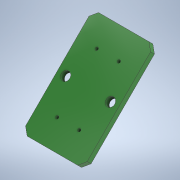
# Autodesk Inventor part: Button Module
Saved by Autodesk Inventor 2020 (Build 240168000, 168)
## iProperties
Created: 2021-01-14
Part Number: Button Module
Material: Generic
Document SubType Name: Modeling
Designer: Luke
Density: 1 g/cm^3
Appearance: Default
Author: Luke
Autodesk Inventor part; units mm, degrees
ref_plane "YZ Plane" through (0, 0, 0) normal (1, 0, 0) x (0, 1, 0)
ref_plane "XZ Plane" through (0, 0, 0) normal (0, 1, 0) x (-1, 0, 0)
ref_plane "XY Plane" through (0, 0, 0) normal (0, 0, 1) x (1, 0, 0)
ref_plane "Work Plane1" through (10.7635, -28.1998, -30.3509) normal (0, -0.7071068, -0.7071068) x (1, 0, 0)
sketch "Sketch1" plane through (10.7635, -28.1998, -30.3509) normal (0, -0.7071068, -0.7071068) x (1, 0, 0)
  line L0 (-49.4847, -25.5492) -> (-49.4847, -5.2292)
  arc A0 (-49.4466, -5.2292) -> (-49.5228, -5.2292) centre (-49.4847, -5.2292) ccw
  arc A1 (-49.5228, -25.5492) -> (-49.4466, -25.5492) centre (-49.4847, -25.5492) ccw
  line L1 (-49.4847, -5.2292) -> (-48.2147, -3.9592)
  arc A2 (-48.1878, -3.9861) -> (-48.2416, -3.9323) centre (-48.2147, -3.9592) ccw
  arc A3 (-49.5116, -5.2023) -> (-49.4578, -5.2561) centre (-49.4847, -5.2292) ccw
  line L2 (-48.2147, -3.9592) -> (-36.7847, -3.9592)
  arc A4 (-36.7847, -3.9973) -> (-36.7847, -3.9211) centre (-36.7847, -3.9592) ccw
  arc A5 (-48.2147, -3.9211) -> (-48.2147, -3.9973) centre (-48.2147, -3.9592) ccw
  line L3 (-36.7847, -3.9592) -> (-35.5147, -5.2292)
  arc A6 (-35.5416, -5.2561) -> (-35.4878, -5.2023) centre (-35.5147, -5.2292) ccw
  arc A7 (-36.7578, -3.9323) -> (-36.8116, -3.9861) centre (-36.7847, -3.9592) ccw
  line L4 (-35.5147, -5.2292) -> (-35.5147, -25.5492)
  arc A8 (-35.5528, -25.5492) -> (-35.4766, -25.5492) centre (-35.5147, -25.5492) ccw
  arc A9 (-35.4766, -5.2292) -> (-35.5528, -5.2292) centre (-35.5147, -5.2292) ccw
  line L5 (-35.5147, -25.5492) -> (-36.7847, -26.8192)
  arc A10 (-36.8116, -26.7923) -> (-36.7578, -26.8461) centre (-36.7847, -26.8192) ccw
  arc A11 (-35.4878, -25.5761) -> (-35.5416, -25.5223) centre (-35.5147, -25.5492) ccw
  line L6 (-36.7847, -26.8192) -> (-48.2147, -26.8192)
  arc A12 (-48.2147, -26.7811) -> (-48.2147, -26.8573) centre (-48.2147, -26.8192) ccw
  arc A13 (-36.7847, -26.8573) -> (-36.7847, -26.7811) centre (-36.7847, -26.8192) ccw
  line L7 (-48.2147, -26.8192) -> (-49.4847, -25.5492)
  arc A14 (-49.4578, -25.5223) -> (-49.5116, -25.5761) centre (-49.4847, -25.5492) ccw
  arc A15 (-48.2416, -26.8461) -> (-48.1878, -26.7923) centre (-48.2147, -26.8192) ccw
  circle A16 centre (-47.5797, -15.3892) radius 0.9525
  circle A17 centre (-37.4197, -15.3892) radius 0.9525
  arc A18 (-39.9597, -8.6572) -> (-39.9597, -9.2612) centre (-39.9597, -8.9592) ccw
  arc A19 (-39.9597, -9.2612) -> (-39.9597, -8.6572) centre (-39.9597, -8.9592) ccw
  arc A20 (-39.9597, -8.6572) -> (-39.9597, -9.2612) centre (-39.9597, -8.9592) ccw
  arc A21 (-39.9597, -9.2612) -> (-39.9597, -8.6572) centre (-39.9597, -8.9592) ccw
  arc A22 (-44.9597, -8.6572) -> (-44.9597, -9.2612) centre (-44.9597, -8.9592) ccw
  arc A23 (-44.9597, -9.2612) -> (-44.9597, -8.6572) centre (-44.9597, -8.9592) ccw
  arc A24 (-44.9597, -8.6572) -> (-44.9597, -9.2612) centre (-44.9597, -8.9592) ccw
  arc A25 (-44.9597, -9.2612) -> (-44.9597, -8.6572) centre (-44.9597, -8.9592) ccw
  arc A26 (-39.9597, -21.3572) -> (-39.9597, -21.9612) centre (-39.9597, -21.6592) ccw
  arc A27 (-39.9597, -21.9612) -> (-39.9597, -21.3572) centre (-39.9597, -21.6592) ccw
  arc A28 (-39.9597, -21.3572) -> (-39.9597, -21.9612) centre (-39.9597, -21.6592) ccw
  arc A29 (-39.9597, -21.9612) -> (-39.9597, -21.3572) centre (-39.9597, -21.6592) ccw
  arc A30 (-44.9597, -21.3572) -> (-44.9597, -21.9612) centre (-44.9597, -21.6592) ccw
  arc A31 (-44.9597, -21.9612) -> (-44.9597, -21.3572) centre (-44.9597, -21.6592) ccw
  arc A32 (-44.9597, -21.3572) -> (-44.9597, -21.9612) centre (-44.9597, -21.6592) ccw
  arc A33 (-44.9597, -21.9612) -> (-44.9597, -21.3572) centre (-44.9597, -21.6592) ccw
  point P0 (-39.9597, -21.9612)
  point P1 (-39.9597, -21.3572)
  point P2 (-39.9597, -9.2612)
  point P3 (-39.9597, -8.6572)
  point P4 (-48.2147, -26.8192)
  point P5 (-36.7847, -26.8192)
  point P6 (-35.5147, -25.5492)
  point P7 (-35.5147, -5.2292)
  point P8 (-36.7847, -3.9592)
  point P9 (-44.9597, -9.2612)
  point P10 (-44.9597, -8.6572)
  point P11 (-44.9597, -21.9612)
  constraints: 64 point on circle, 34 centre point, 16 end point
extrude "Extrusion1" add sketch "Sketch1" along normal blind 1.23 contours L0 L1 L2 L3 L4 L5 L6 L7
ref_plane "Work Plane2" through (-31.7362, -24.5021, -34.0485) normal (1, 0, 0) x (0, -0.7071068, -0.7071068)
ref_plane "Work Plane3" through (-26.0212, -17.3179, -41.2327) normal (0, 0.7071068, -0.7071068) x (-1, 0, 0)
ref_plane "Work Plane4" through (-37.4512, -10.1054, -50.1847) normal (0, 0, -1) x (1, 0, 0)
ref_plane "Work Plane5" through (-26.0212, -17.3179, -41.2327) normal (0, 0.7071068, -0.7071068) x (-1, 0, 0)
body "Solid1"
